Autodesk Fusion 360 part; units mm, degrees
note: some values were not read from the file. Chosen so that the rebuilt part matches the saved one: which bodies a step acts on; which face or edge a step refers to. Set by a fixed rule: which sketch regions a step uses.
(part 2 of 2)
move_body "Move52" bodies 3 to x (1, 0, 0) y (0, 1, 0) z (0, 0, 1) at (0, 40, 0)
move_body "Move53" bodies 1 to x (1, 0, 0) y (0, 1, 0) z (0, 0, 1) at (0, 60, 0)
move_body "Move54" bodies 2 to x (1, 0, 0) y (0, 1, 0) z (0, 0, 1) at (0, -10, 0)
move_body "Move55" bodies 5 to x (1, 0, 0) y (0, 1, 0) z (0, 0, 1) at (200, 0, 0)
extrude "Extrude84" add sketch "Readout-Holder" along normal blind 1.6 from surface at 32 contours A58 A61 A67 | A58 A67 | A58 A69 | A58 A61 A69 | A61 A63 A69 | A58 A61 A68 | A58 A68 | A61 A63 A67 | A63 A69 A72 | A61 A63 A68 | A63 A67 A70 | A63 A67 A70 | A63 A69 A72 | A69 A72 | A63 A68 A71 | A67 A70 | A63 A68 A71 | A68 A71 picked at (228.0054, -16.1689) picked at (200, 32.3378) picked at (171.9946, -16.1689) bodies 5
extrude "Extrude85" add sketch "Readout-Holder" against normal blind 1 from surface at 20 contours A69 A72 | A69 A72 | A67 A70 | A67 A70 | A68 A71 | A68 A71 bodies 5
extrude "Extrude86" add 3 faces at (199.9258, 19, -31.2216) (227.4125, 19, 16.1446) (172.213, 19, 16.7784) along direction (0, -1, 0) blind 0.6 on bodies 5 bodies 5
move_body "Move56" bodies 5 to x (1, 0, 0) y (0, 1, 0) z (0, 0, 1) at (-200, 0, 0)
move_body "Move57" bodies 1 to x (1, 0, 0) y (0, 1, 0) z (0, 0, 1) at (0, -10, 0)
move_body "Move58" bodies 5 to x (1, 0, 0) y (0, 1, 0) z (0, 0, 1) at (0, -20, 0)
sketch "Ring.Gem.Support" plane through (0, 0, 0) normal (0, 1, 0) x (1, 0, 0)
  circle A0 centre (0, 0) radius 30
  circle A1 centre (0, 0) radius 40
  line L0 (0, 0) -> (0, 35) construction
  circle A2 centre (0, 35) radius 3.175
  circle A3 centre (-30.3109, -17.5) radius 3.175
  circle A4 centre (30.3109, -17.5) radius 3.175
  dimension "d413" = 60
  dimension "d414" = 80
  dimension "d424" = 35
  dimension "d425" = 6.35
  dimension "d427" = 360
  constraint coincident A0.centre A1.centre
  constraint vertical L0
  constraint coincident L0.end A2.centre
  measures "d413" diameter of A0
  measures "d414" diameter of A1
  measures "d424" distance of A0.centre L0.end
  measures "d425" diameter of A2
extrude "Extrude87" add sketch "Ring.Gem.Support" along normal blind 2.86 separate body contours A1 | A2 | A3 | A4 makes body 20
move_body "Move59" bodies 20 to x (1, 0, 0) y (0, 1, 0) z (0, 0, 1) at (0, 70, 0)
extrude "Extrude89" cut sketch "Ring.Gem.Support" along normal blind 82 contours A2 | A3 | A4 bodies 20
sketch "PCB.Plates" plane through (0, 0, 0) normal (0, 1, 0) x (1, 0, 0)
  circle A0 centre (0, 0) radius 30
  circle A1 centre (0, 0) radius 40
  line L0 (0, 0) -> (0, 35) construction
  circle A2 centre (0, 35) radius 3
  circle A3 centre (-30.3109, -17.5) radius 3
  circle A4 centre (30.3109, -17.5) radius 3
  circle A5 centre (0, 0) radius 32 construction
  circle A6 centre (0, 0) radius 34
  circle A7 centre (0, 32) radius 1
  circle A8 centre (-27.7128, -16) radius 1
  circle A9 centre (27.7128, -16) radius 1
  dimension "d430" = 60
  dimension "d431" = 80
  dimension "d432" = 35
  dimension "d434" = 6
  dimension "d436" = 360
  dimension "d437" = 64
  dimension "d438" = 68
  dimension "d439" = 2
  dimension "d441" = 360
  constraint coincident A0.centre A1.centre
  constraint vertical L0
  constraint coincident L0.end A2.centre
  constraint concentric A1 A5
  constraint concentric A5 A6
  constraint coincident A2 A7.centre
  constraint coincident A5 A7.centre
  measures "d430" diameter of A0
  measures "d431" diameter of A1
  measures "d432" distance of A0.centre L0.end
  measures "d434" diameter of A2
  measures "d437" diameter of A5
  measures "d438" diameter of A6
  measures "d439" diameter of A7
move_body "Move60" bodies 5 to x (1, 0, 0) y (0, 1, 0) z (0, 0, 1) at (0, 4, 0)
extrude "Extrude90" add sketch "PCB.Plates" along normal blind 1.6 separate body contours A0 | A1 | A2 A3 A4 A6 A7 A8 A9 | A2 A7 | A3 A8 | A4 A9 picked at (-0.0039, 31.6712) picked at (-27.4352, -15.8236) picked at (27.428, -15.8356) makes body 21
move_body "Move61" bodies 21 to x (1, 0, 0) y (0, 1, 0) z (0, 0, 1) at (0, 24, 0)
extrude "Extrude91" add sketch "PCB.Plates" along normal blind 1.6 separate body contours A2 A6 A7 | A2 A3 A4 A6 A7 A8 A9 | A3 A6 A8 | A4 A6 A9 makes body 22
extrude "Extrude92" add sketch "PCB.Plates" along normal blind 1.6 contours A0 bodies 22
move_body "Move62" bodies 22 to x (1, 0, 0) y (0, 1, 0) z (0, 0, 1) at (0, 2, 0)
move_body "Move63" bodies 22 to x (1, 0, 0) y (0, 1, 0) z (0, 0, 1) at (0, 0.4, 0)
move_body "Move64" bodies 21 to x (1, 0, 0) y (0, 1, 0) z (0, 0, 1) at (0, -8, 0)
move_body "Move74" bodies 5 21 22 to x (1, 0, 0) y (0, 1, 0) z (0, 0, 1) at (0, -2, 0)
move_body "Move75" bodies 22 5 21 to x (1, 0, 0) y (0, 1, 0) z (0, 0, 1) at (0, -2, 0)
extrude "Extrude93" add sketch "PCB.Plates" along normal blind 0.7 separate body contours A1 | A2 A3 A4 A6 A7 A8 A9 | A2 A7 | A3 A8 | A4 A9 picked at (-0.0039, 31.6712) picked at (-27.4352, -15.8236) picked at (27.428, -15.8356) makes body 23
extrude "Extrude95" add sketch "PCB.Plates" along normal blind 0.7 contours A0 bodies 23
move_body "Move76" bodies 23 to x (1, 0, 0) y (0, 1, 0) z (0, 0, 1) at (0, 16, 0)
move_body "Move79" bodies 20 to x (1, 0, 0) y (0, 1, 0) z (0, 0, 1) at (0, -45, 0)
move_body "Move80" bodies 20 to x (1, 0, 0) y (0, 1, 0) z (0, 0, 1) at (0, -1.4, 0)
pattern_linear "R-Pattern1" count 9 spacing 12.875 along (0, 1, 0) of bodies 20 makes body 24 at (36.4061, 36.475, 3.4777) makes body 25 at (36.4061, 49.35, 3.4777) makes body 26 at (36.4061, 62.225, 3.4777) makes body 27 at (36.4061, 75.1, 3.4777) makes body 28 at (36.4061, 87.975, 3.4777) makes body 29 at (36.4061, 100.85, 3.4777) makes body 30 at (36.4061, 113.725, 3.4777) makes body 31 at (36.4061, 126.6, 3.4777)
extrude "Extrude97" add sketch "PCB.Plates" along normal blind 150 separate body contours A2 A6 | A2 A6 A7 | A2 A7 | A3 A6 | A3 A6 A8 | A3 A8 | A4 A6 A9 | A4 A6 | A4 A9 picked at (0.0246, 32.3369) picked at (-28.0169, -16.1472) picked at (27.9931, -16.1885) makes body 32 at (2.9851, 100, -35.2987) makes body 33 at (33.296, 100, 17.2013) makes body 34 at (-27.3258, 100, 17.2013)
extrude "Extrude98" cut 3 faces at (-31.9248, 0, 16.8882) (30.2718, 0, 16.8718) (-0.5, 0, -33.2662) along direction (0, 1, 0) blind 11 on bodies 32 33 34 bodies 32 33 34
move_body "Move83" bodies 25 23 24 28 30 27 33 31 26 20 29 34 32 to x (1, 0, 0) y (0, 1, 0) z (0, 0, 1) at (0, 10, 0)
move_body "Move84" bodies 22 to x (1, 0, 0) y (0, 1, 0) z (0, 0, 1) at (0, -4, 0)
extrude "Extrude99" add 3 faces at (-0.3003, -1.6, -32.1446) (27.6386, -1.6, 16.7784) (-27.787, -1.6, 16.7784) along direction (0, -1, 0) blind 4 separate body on bodies 5 makes body 35 at (28.7078, -4.2667, 16.0996) makes body 36 at (-0.9397, -4.2667, -32.342) makes body 37 at (-26.7178, -4.2667, 16.0996)
combine "Combine6" operation add target body 5 tool bodies 37 36 35
extrude "Extrude100" add 1 faces at (20.9098, 0, -17.9888) along direction (0, -1, 0) blind 4 on bodies 5 bodies 5
extrude "Extrude101" cut 1 faces at (33.5401, 2, -1.6891) along direction (0, -1, 0) blind 1 from surface at 3 on bodies 5 bodies 5
extrude "Extrude102" add 1 faces at (-59.5986, 0, 11.2919) along direction (0, -1, 0) blind 4 on bodies 4 bodies 4
sketch "Screenshot.Cutter" plane through (0, 0, 0) normal (1, 0, 0) x (0, 0, -1)
  line L0 (0, 0) -> (-118.2102, 0)
  line L1 (-118.2102, 0) -> (-118.2102, 173.4447)
  line L2 (-118.2102, 173.4447) -> (0, 173.4447)
  line L3 (0, 173.4447) -> (0, 0)
  line L4 (-118.2102, 0) -> (0, 0)
  line L5 (0, 0) -> (0, -24.6458)
  line L6 (0, -24.6458) -> (-118.2102, -24.6458)
  line L7 (-118.2102, -24.6458) -> (-118.2102, 0)
  constraint horizontal L0
  constraint vertical L1
  constraint horizontal L2
  constraint vertical L3
  constraint coincident L0.start L3.end
  constraint horizontal L4
  constraint vertical L5
  constraint horizontal L6
  constraint vertical L7
extrude "Extrude103" cut 14 faces at (-44.2674, 10, 0.226) (-41.2762, 10, 19.2988) (-27.3244, 10, 34.9564) (-9.2808, 10, 43.6458) (10.746, 10, 43.6458) (28.7896, 10, 34.9564) (39.811, 10, 19.2988) (45.7326, 10, 0.226) (39.811, 10, -19.7507) (28.7896, 10, -35.4084) (10.746, 10, -44.0977) (-9.2808, 10, -44.0977) (-27.3244, 10, -35.4084) (-41.2762, 10, -19.7507) along direction (0, 1, 0) blind 8 on bodies 5 bodies 5
extrude "Extrude104" add sketch "Vessel.Base" against normal blind 4 contours A34 | A35 | A36 | A37 | A38 | A39 | A40 | A41 | A42 | A43 | A44 | A45 | A46 | A47 bodies 4
extrude "Extrude105" add 1 faces at (-35.0312, 5, 7.1014) along direction (0, 1, 0) blind 1 on bodies 4 bodies 4
extrude "Extrude107" cut sketch "Vessel.Base" along normal blind 1 from surface at 5 contours A55 bodies 4
extrude "Extrude108" add 1 faces at (35.3926, 6, 14.9074) along direction (0, -1, 0) blind 1 on bodies 4 bodies 4
extrude "Extrude109" cut 1 faces at (35.3926, 6, 14.9074) along direction (0, -1, 0) blind 2 on bodies 4 bodies 4
extrude "Extrude110" add 1 faces at (35.3926, 4, 14.9074) along direction (0, 1, 0) blind 1 on bodies 4 bodies 4
extrude "Extrude111" cut 1 faces at (-46.5501, 11, 16.9583) along direction (0, 1, 0) blind 1 on bodies 5 bodies 5
extrude "Extrude112" cut 1 faces at (-46.5501, 8, 16.9583) along direction (0, 1, 0) blind 1 on bodies 5 bodies 5
extrude "Extrude113" add 1 faces at (-46.5501, 7, 16.9583) along direction (0, 1, 0) blind 1 on bodies 5 bodies 5
extrude "Extrude114" add 1 faces at (-46.5501, 10, 16.9583) along direction (0, 1, 0) blind 1 on bodies 5 bodies 5
extrude "Extrude106" [suppressed]
named bodies: "Sup.Ring.1", "Cylinder.Wall", "Sup.Ring.2", "Vessel.Base", "Readout.Support", "Door.Sup.A.Inner.B", "Door.Inner.Support", "Door.Sup.B.Outer.B", "Door.Outer.Support", "Door.Bes.A.Inner", "Door.Bes.B.Outer", "Door", "Handle.1", "Handle.2", "E.Ring.9", "Readout.Adapter.I", "Readout.Adapter.O", "ThGEM", "E.Ring.8", "E.Ring.7", "E.Ring.6", "E.Ring.5", "E.Ring.4", "E.Ring.3", "E.Ring.2", "E.Ring.1", "Holder.1", "Holder.2", "Holder.3"
